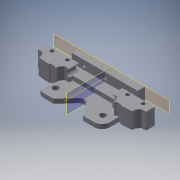
# Autodesk Inventor part: bumper lever support
Saved by Autodesk Inventor 2016 (Build 200138000, 138)
## iProperties
Created: 2015-09-30
Part Number: bumper lever support
Material: Generic
Document SubType Name: Modeling
Designer: Jesse Stevenson
Density: 1 g/cm^3
Appearance: Default
Author: Jesse Stevenson
Autodesk Inventor part; units mm, degrees
ref_plane "YZ Plane" through (0, 0, 0) normal (1, 0, 0) x (0, 1, 0)
ref_plane "XZ Plane" through (0, 0, 0) normal (0, 1, 0) x (-1, 0, 0)
ref_plane "XY Plane" through (0, 0, 0) normal (0, 0, 1) x (1, 0, 0)
ref_plane "Work Plane1" through (-0.2015, 0, 0) normal (0, 0, 1) x (1, 0, 0)
sketch "Sketch1" plane through (-0.2015, 0, 0) normal (0, 0, 1) x (1, 0, 0)
  circle A0 centre (19.4801, 3.175) radius 1.0541 projected
  circle A1 centre (44.8801, 3.175) radius 1.0541 projected
  circle A2 centre (57.5801, 3.175) radius 1.0541 construction
  circle A3 centre (6.7801, 3.175) radius 1.0541 construction
  circle A4 centre (32.1801, 3.175) radius 1.0541 projected
  line L0 (0.2015, 0) -> (64.1587, 0) construction
  line L1 (64.1587, 0) -> (64.1587, 6.35) construction
  line L2 (0.2015, 6.35) -> (64.1587, 6.35) construction
  line L3 (0.2015, 0) -> (0.2015, 6.35) construction
  line L4 (52.3672, 6.35) -> (11.9931, 6.35)
  line L5 (11.9931, 6.35) -> (11.9931, 0)
  line L6 (11.9931, 0) -> (52.3672, 0)
  line L7 (52.3672, 0) -> (52.3672, 6.35)
  line L8 (44.8801, 3.175) -> (52.3672, 3.175) construction
  line L9 (19.4801, 3.175) -> (11.9931, 3.175) construction
  constraints: 12 end point, 2 midpoint, 2 parallel, 2 point on line, 1 collinear, 1 horizontal, 1 perpendicular
extrude "Extrusion1" add sketch "Sketch1" along normal blind 4.318
sketch "Sketch2" plane through (11.7916, 0, 0) normal (0, -1, 0) x (1, 0, 0)
  line L0 (0, 0) -> (40.3741, 0) projected
  line L1 (40.3741, 0) -> (40.3741, 4.318) projected
  line L2 (0, 4.318) -> (40.3741, 4.318) projected
  line L3 (0, 0) -> (0, 4.318) projected
  point P0 (-11.7916, 0)
extrude "Extrusion2" add sketch "Sketch2" along normal blind 4.318
sketch "Sketch3" plane through (-0.2015, 0, 4.318) normal (0, 0, 1) x (1, 0, 0)
  line L0 (52.3672, 6.35) -> (52.3672, -4.318) projected
  line L1 (52.3672, 1.016) -> (11.9931, 1.016)
  line L2 (11.9931, 6.35) -> (11.9931, -4.318) projected
  line L3 (52.3672, -4.318) -> (11.9931, -4.318) projected
  line L4 (52.3672, 1.016) -> (11.9931, 1.016)
  line L5 (11.9931, 1.016) -> (11.9931, -4.318)
  line L6 (11.9931, -4.318) -> (52.3672, -4.318)
  line L7 (52.3672, -4.318) -> (52.3672, 1.016)
  point P0 (0.2015, 0)
  constraints: 10 end point, 2 midpoint, 2 parallel, 1 horizontal, 1 perpendicular
extrude "Extrusion3" add sketch "Sketch3" along normal blind 21.7805
sketch "Sketch4" plane through (11.7916, -4.318, 0) normal (0, -1, 0) x (1, 0, 0)
  line L0 (0, 0) -> (40.3741, 0) construction
  line L1 (40.3741, 0) -> (40.3741, 26.0985) construction
  line L2 (0, 26.0985) -> (40.3741, 26.0985) construction
  line L3 (0, 0) -> (0, 26.0985) construction
  line L4 (0, 26.0985) -> (40.3741, 26.0985) construction
  line L5 (28.8565, 26.0985) -> (22.9541, 18.3371)
  line L6 (18.0716, 18.1299) -> (10.868, 26.0985)
  line L7 (25.9053, 22.2178) -> (20.1871, 22.2178) construction
  line L8 (20.1871, 22.2178) -> (20.1871, 26.0985) construction
  line L9 (20.1871, 22.2178) -> (14.4698, 22.1142) construction
  line L10 (10.868, 26.0985) -> (28.8565, 26.0985)
  arc A0 (18.0716, 18.1299) -> (22.9541, 18.3371) centre (20.4268, 20.259) ccw
  point P0 (-11.7916, 0)
  point P1 (20.6377, 15.2912)
  dimension "d8" = 3.175
  constraints: 12 end point, 4 point on line, 3 midpoint, 2 point on circle, 2 tangent, 1 centre point, 1 collinear, 1 equal length, 1 horizontal, 1 vertical
  measures "d8" radius of A0
extrude "Extrusion4" cut sketch "Sketch4" against normal through all
sketch "Sketch5" plane through (11.7916, -4.318, 0) normal (0, -1, 0) x (1, 0, 0)
  line L0 (28.8565, 26.0985) -> (22.9541, 18.3371) projected
  arc A0 (18.0716, 18.1299) -> (22.9541, 18.3371) centre (20.4268, 20.259) ccw projected
  line L1 (18.0716, 18.1299) -> (10.868, 26.0985) projected
  line L2 (0, 26.0985) -> (10.868, 26.0985) projected
  line L3 (0, 0) -> (0, 26.0985) projected
  line L4 (0, 0) -> (40.3741, 0) projected
  line L5 (40.3741, 0) -> (40.3741, 26.0985) projected
  line L6 (28.8565, 26.0985) -> (40.3741, 26.0985) projected
  line L7 (40.3741, 0) -> (40.3741, 26.0985) construction
  line L8 (0, 4.318) -> (0, 26.0985) construction
  line L9 (40.3741, 19.7485) -> (0, 19.7485) construction
  line L10 (5.7588, 24.0238) -> (5.7588, 16.2202) construction
  line L11 (28.8565, 26.0985) -> (40.3741, 26.0985) construction
  line L12 (34.6153, 26.0985) -> (34.6153, 15.2083) construction
  line L13 (34.6153, 22.1235) -> (40.3741, 22.1235) construction
  line L14 (40.3741, 4.318) -> (40.3741, 26.0985) construction
  line L15 (5.7588, 22.1235) -> (0, 22.1235) construction
  line L16 (0, 0) -> (0, 26.0985) construction
  circle A1 centre (34.6153, 19.7485) radius 1.7859
  circle A2 centre (5.7588, 19.7485) radius 1.7859
  point P0 (-11.7916, 0)
  dimension "d10" = 6.35
  dimension "d16" = 3.5719
  constraints: 11 point on line, 10 end point, 3 perpendicular, 2 centre point, 2 vertical, 1 collinear, 1 equal radius, 1 midpoint
  measures "d10" distance between parallel lines of L2 L9
  measures "d16" diameter of A1
extrude "Extrusion5" cut sketch "Sketch5" against normal through all contours A1 | A2
sketch "Sketch6" plane through (-0.2015, 0, 26.0985) normal (0, 0, 1) x (1, 0, 0)
  line L0 (11.9931, 1.016) -> (11.9931, -4.318) construction
  line L1 (52.3672, -4.318) -> (52.3672, 1.016) construction
  circle A0 centre (32.1801, 3.175) radius 1.0541 construction
  circle A1 centre (44.8801, 3.175) radius 1.0541 construction
  circle A2 centre (19.4801, 3.175) radius 1.0541 construction
  line L2 (52.3672, 6.35) -> (11.9931, 6.35) construction
  line L3 (52.3672, 6.35) -> (52.3672, -4.318) construction
  line L4 (11.9931, -4.318) -> (52.3672, -4.318) construction
  line L5 (11.9931, 6.35) -> (11.9931, -4.318) construction
  line L6 (52.3672, -1.651) -> (11.9931, -1.651)
  line L7 (52.3672, -1.651) -> (11.9931, -1.651)
  line L8 (11.9931, -1.651) -> (11.9931, 6.35)
  line L9 (11.9931, 6.35) -> (52.3672, 6.35)
  line L10 (52.3672, 6.35) -> (52.3672, -1.651)
  point P0 (0.2015, 0)
  constraints: 10 end point, 2 parallel, 2 perpendicular, 2 point on line, 1 horizontal
extrude "Extrusion6" cut sketch "Sketch6" against normal blind 15.4305
fillet "Fillet1" radius 4.7625 3 edges at (11.7916, -2.9845, 26.0985) (11.7916, -1.651, 18.3833) (52.1657, -2.9845, 26.0985)
body "Solid1"
